Autodesk Fusion 360 part; units mm, degrees
(part 3 of 4)
sketch "草图57" plane through (0, 12.5, 0) normal (0, 1, 0) x (-1, 0, 0)
  circle A0 centre (-311.895, -3.8697) radius 1.7
  circle A1 centre (-109.895, -3.8697) radius 1.7
  circle A2 centre (-7.0941, -106.12) radius 1.7
  circle A3 centre (-7.0941, -3.8697) radius 1.7
  circle A4 centre (-210.895, -3.8697) radius 1.7
  circle A5 centre (-311.895, -106.12) radius 1.7
  circle A6 centre (-210.895, -106.12) radius 1.1
  circle A7 centre (-109.895, -106.12) radius 1.1
  arc A8 (-12.4713, -23.8643) -> (-11.9713, -23.3643) centre (-12.4713, -23.3643) ccw
  line L0 (-12.4713, -23.8643) -> (-25.4713, -23.8643)
  arc A9 (-25.9713, -23.3643) -> (-25.4713, -23.8643) centre (-25.4713, -23.3643) ccw
  line L1 (-25.9713, -23.3643) -> (-25.9713, -10.3643)
  arc A10 (-25.4713, -9.8643) -> (-25.9713, -10.3643) centre (-25.4713, -10.3643) ccw
  line L2 (-25.4713, -9.8643) -> (-12.4713, -9.8643)
  arc A11 (-11.9713, -10.3643) -> (-12.4713, -9.8643) centre (-12.4713, -10.3643) ccw
  line L3 (-11.9713, -10.3643) -> (-11.9713, -23.3643)
  arc A12 (-186.3026, -42.9143) -> (-185.8026, -42.4143) centre (-186.3026, -42.4143) ccw
  line L4 (-186.3026, -42.9143) -> (-199.3026, -42.9143)
  arc A13 (-199.8026, -42.4143) -> (-199.3026, -42.9143) centre (-199.3026, -42.4143) ccw
  line L5 (-199.8026, -42.4143) -> (-199.8026, -29.4143)
  arc A14 (-199.3026, -28.9143) -> (-199.8026, -29.4143) centre (-199.3026, -29.4143) ccw
  line L6 (-199.3026, -28.9143) -> (-186.3026, -28.9143)
  arc A15 (-185.8026, -29.4143) -> (-186.3026, -28.9143) centre (-186.3026, -29.4143) ccw
  line L7 (-185.8026, -29.4143) -> (-185.8026, -42.4143)
  arc A16 (-295.8401, -61.9643) -> (-295.3401, -61.4643) centre (-295.8401, -61.4643) ccw
  line L8 (-295.8401, -61.9643) -> (-308.8401, -61.9643)
  arc A17 (-309.3401, -61.4643) -> (-308.8401, -61.9643) centre (-308.8401, -61.4643) ccw
  line L9 (-309.3401, -61.4643) -> (-309.3401, -48.4643)
  arc A18 (-308.8401, -47.9643) -> (-309.3401, -48.4643) centre (-308.8401, -48.4643) ccw
  line L10 (-308.8401, -47.9643) -> (-295.8401, -47.9643)
  arc A19 (-295.3401, -48.4643) -> (-295.8401, -47.9643) centre (-295.8401, -48.4643) ccw
  line L11 (-295.3401, -48.4643) -> (-295.3401, -61.4643)
  line L12 (-128.6526, -29.4143) -> (-128.6526, -42.4143)
  arc A20 (-129.1526, -42.9143) -> (-128.6526, -42.4143) centre (-129.1526, -42.4143) ccw
  line L13 (-129.1526, -42.9143) -> (-142.1526, -42.9143)
  arc A21 (-142.6526, -42.4143) -> (-142.1526, -42.9143) centre (-142.1526, -42.4143) ccw
  line L14 (-142.6526, -42.4143) -> (-142.6526, -29.4143)
  arc A22 (-142.1526, -28.9143) -> (-142.6526, -29.4143) centre (-142.1526, -29.4143) ccw
  line L15 (-142.1526, -28.9143) -> (-129.1526, -28.9143)
  arc A23 (-128.6526, -29.4143) -> (-129.1526, -28.9143) centre (-129.1526, -29.4143) ccw
  arc A24 (-162.4901, -100.0643) -> (-161.9901, -99.5643) centre (-162.4901, -99.5643) ccw
  line L16 (-162.4901, -100.0643) -> (-175.4901, -100.0643)
  arc A25 (-175.9901, -99.5643) -> (-175.4901, -100.0643) centre (-175.4901, -99.5643) ccw
  line L17 (-175.9901, -99.5643) -> (-175.9901, -86.5643)
  arc A26 (-175.4901, -86.0643) -> (-175.9901, -86.5643) centre (-175.4901, -86.5643) ccw
  line L18 (-175.4901, -86.0643) -> (-162.4901, -86.0643)
  arc A27 (-161.9901, -86.5643) -> (-162.4901, -86.0643) centre (-162.4901, -86.5643) ccw
  line L19 (-161.9901, -86.5643) -> (-161.9901, -99.5643)
  arc A28 (-72.0026, -42.9143) -> (-71.5026, -42.4143) centre (-72.0026, -42.4143) ccw
  line L20 (-72.0026, -42.9143) -> (-85.0026, -42.9143)
  arc A29 (-85.5026, -42.4143) -> (-85.0026, -42.9143) centre (-85.0026, -42.4143) ccw
  line L21 (-85.5026, -42.4143) -> (-85.5026, -29.4143)
  arc A30 (-85.0026, -28.9143) -> (-85.5026, -29.4143) centre (-85.0026, -29.4143) ccw
  line L22 (-85.0026, -28.9143) -> (-72.0026, -28.9143)
  arc A31 (-71.5026, -29.4143) -> (-72.0026, -28.9143) centre (-72.0026, -29.4143) ccw
  line L23 (-71.5026, -29.4143) -> (-71.5026, -42.4143)
  arc A32 (-295.8401, -42.9143) -> (-295.3401, -42.4143) centre (-295.8401, -42.4143) ccw
  line L24 (-295.8401, -42.9143) -> (-308.8401, -42.9143)
  arc A33 (-309.3401, -42.4143) -> (-308.8401, -42.9143) centre (-308.8401, -42.4143) ccw
  line L25 (-309.3401, -42.4143) -> (-309.3401, -29.4143)
  arc A34 (-308.8401, -28.9143) -> (-309.3401, -29.4143) centre (-308.8401, -29.4143) ccw
  line L26 (-308.8401, -28.9143) -> (-295.8401, -28.9143)
  arc A35 (-295.3401, -29.4143) -> (-295.8401, -28.9143) centre (-295.8401, -29.4143) ccw
  line L27 (-295.3401, -29.4143) -> (-295.3401, -42.4143)
  arc A36 (-256.4458, -60.9643) -> (-255.9458, -60.4643) centre (-256.4458, -60.4643) ccw
  line L28 (-256.4458, -60.9643) -> (-262.4458, -60.9643)
  arc A37 (-262.9458, -60.4643) -> (-262.4458, -60.9643) centre (-262.4458, -60.4643) ccw
  line L29 (-262.9458, -60.4643) -> (-262.9458, -46.4643)
  arc A38 (-262.4458, -45.9643) -> (-262.9458, -46.4643) centre (-262.4458, -46.4643) ccw
  line L30 (-262.4458, -45.9643) -> (-256.4458, -45.9643)
  arc A39 (-255.9458, -46.4643) -> (-256.4458, -45.9643) centre (-256.4458, -46.4643) ccw
  line L31 (-255.9458, -46.4643) -> (-255.9458, -60.4643)
  arc A40 (-110.1026, -42.9143) -> (-109.6026, -42.4143) centre (-110.1026, -42.4143) ccw
  line L32 (-110.1026, -42.9143) -> (-123.1026, -42.9143)
  arc A41 (-123.6026, -42.4143) -> (-123.1026, -42.9143) centre (-123.1026, -42.4143) ccw
  line L33 (-123.6026, -42.4143) -> (-123.6026, -29.4143)
  arc A42 (-123.1026, -28.9143) -> (-123.6026, -29.4143) centre (-123.1026, -29.4143) ccw
  line L34 (-123.1026, -28.9143) -> (-110.1026, -28.9143)
  arc A43 (-109.6026, -29.4143) -> (-110.1026, -28.9143) centre (-110.1026, -29.4143) ccw
  line L35 (-109.6026, -29.4143) -> (-109.6026, -42.4143)
  line L36 (-52.4526, -29.4143) -> (-52.4526, -42.4143)
  arc A44 (-52.9526, -42.9143) -> (-52.4526, -42.4143) centre (-52.9526, -42.4143) ccw
  line L37 (-52.9526, -42.9143) -> (-65.9526, -42.9143)
  arc A45 (-66.4526, -42.4143) -> (-65.9526, -42.9143) centre (-65.9526, -42.4143) ccw
  line L38 (-66.4526, -42.4143) -> (-66.4526, -29.4143)
  arc A46 (-65.9526, -28.9143) -> (-66.4526, -29.4143) centre (-65.9526, -29.4143) ccw
  line L39 (-65.9526, -28.9143) -> (-52.9526, -28.9143)
  arc A47 (-52.4526, -29.4143) -> (-52.9526, -28.9143) centre (-52.9526, -29.4143) ccw
  arc A48 (-148.2026, -42.9143) -> (-147.7026, -42.4143) centre (-148.2026, -42.4143) ccw
  line L40 (-148.2026, -42.9143) -> (-161.2026, -42.9143)
  arc A49 (-161.7026, -42.4143) -> (-161.2026, -42.9143) centre (-161.2026, -42.4143) ccw
  line L41 (-161.7026, -42.4143) -> (-161.7026, -29.4143)
  arc A50 (-161.2026, -28.9143) -> (-161.7026, -29.4143) centre (-161.2026, -29.4143) ccw
  line L42 (-161.2026, -28.9143) -> (-148.2026, -28.9143)
  arc A51 (-147.7026, -29.4143) -> (-148.2026, -28.9143) centre (-148.2026, -29.4143) ccw
  line L43 (-147.7026, -29.4143) -> (-147.7026, -42.4143)
  arc A52 (-282.7031, -99.0643) -> (-282.2031, -98.5643) centre (-282.7031, -98.5643) ccw
  line L44 (-282.7031, -99.0643) -> (-288.7031, -99.0643)
  arc A53 (-289.2031, -98.5643) -> (-288.7031, -99.0643) centre (-288.7031, -98.5643) ccw
  line L45 (-289.2031, -98.5643) -> (-289.2031, -84.5643)
  arc A54 (-288.7031, -84.0643) -> (-289.2031, -84.5643) centre (-288.7031, -84.5643) ccw
  line L46 (-288.7031, -84.0643) -> (-282.7031, -84.0643)
  arc A55 (-282.2031, -84.5643) -> (-282.7031, -84.0643) centre (-282.7031, -84.5643) ccw
  line L47 (-282.2031, -84.5643) -> (-282.2031, -98.5643)
  arc A56 (-23.5901, -99.5643) -> (-23.0901, -100.0643) centre (-23.0901, -99.5643) ccw
  line L48 (-23.5901, -99.5643) -> (-23.5901, -86.5643)
  arc A57 (-23.0901, -86.0643) -> (-23.5901, -86.5643) centre (-23.0901, -86.5643) ccw
  line L49 (-23.0901, -86.0643) -> (-10.0901, -86.0643)
  arc A58 (-9.5901, -86.5643) -> (-10.0901, -86.0643) centre (-10.0901, -86.5643) ccw
  line L50 (-9.5901, -86.5643) -> (-9.5901, -99.5643)
  arc A59 (-10.0901, -100.0643) -> (-9.5901, -99.5643) centre (-10.0901, -99.5643) ccw
  line L51 (-10.0901, -100.0643) -> (-23.0901, -100.0643)
  arc A60 (-60.0963, -23.8643) -> (-59.5963, -23.3643) centre (-60.0963, -23.3643) ccw
  line L52 (-60.0963, -23.8643) -> (-73.0963, -23.8643)
  arc A61 (-73.5963, -23.3643) -> (-73.0963, -23.8643) centre (-73.0963, -23.3643) ccw
  line L53 (-73.5963, -23.3643) -> (-73.5963, -10.3643)
  arc A62 (-73.0963, -9.8643) -> (-73.5963, -10.3643) centre (-73.0963, -10.3643) ccw
  line L54 (-73.0963, -9.8643) -> (-60.0963, -9.8643)
  arc A63 (-59.5963, -10.3643) -> (-60.0963, -9.8643) centre (-60.0963, -10.3643) ccw
  line L55 (-59.5963, -10.3643) -> (-59.5963, -23.3643)
  arc A64 (-181.5401, -100.0643) -> (-181.0401, -99.5643) centre (-181.5401, -99.5643) ccw
  line L56 (-181.5401, -100.0643) -> (-194.5401, -100.0643)
  arc A65 (-195.0401, -99.5643) -> (-194.5401, -100.0643) centre (-194.5401, -99.5643) ccw
  line L57 (-195.0401, -99.5643) -> (-195.0401, -86.5643)
  arc A66 (-194.5401, -86.0643) -> (-195.0401, -86.5643) centre (-194.5401, -86.5643) ccw
  line L58 (-194.5401, -86.0643) -> (-181.5401, -86.0643)
  arc A67 (-181.0401, -86.5643) -> (-181.5401, -86.0643) centre (-181.5401, -86.5643) ccw
  line L59 (-181.0401, -86.5643) -> (-181.0401, -99.5643)
  arc A68 (-105.3401, -100.0643) -> (-104.8401, -99.5643) centre (-105.3401, -99.5643) ccw
  line L60 (-105.3401, -100.0643) -> (-118.3401, -100.0643)
  arc A69 (-118.8401, -99.5643) -> (-118.3401, -100.0643) centre (-118.3401, -99.5643) ccw
  line L61 (-118.8401, -99.5643) -> (-118.8401, -86.5643)
  arc A70 (-118.3401, -86.0643) -> (-118.8401, -86.5643) centre (-118.3401, -86.5643) ccw
  line L62 (-118.3401, -86.0643) -> (-105.3401, -86.0643)
  arc A71 (-104.8401, -86.5643) -> (-105.3401, -86.0643) centre (-105.3401, -86.5643) ccw
  line L63 (-104.8401, -86.5643) -> (-104.8401, -99.5643)
  arc A72 (-131.5338, -23.8643) -> (-131.0338, -23.3643) centre (-131.5338, -23.3643) ccw
  line L64 (-131.5338, -23.8643) -> (-144.5338, -23.8643)
  arc A73 (-145.0338, -23.3643) -> (-144.5338, -23.8643) centre (-144.5338, -23.3643) ccw
  line L65 (-145.0338, -23.3643) -> (-145.0338, -10.3643)
  arc A74 (-144.5338, -9.8643) -> (-145.0338, -10.3643) centre (-144.5338, -10.3643) ccw
  line L66 (-144.5338, -9.8643) -> (-131.5338, -9.8643)
  arc A75 (-131.0338, -10.3643) -> (-131.5338, -9.8643) centre (-131.5338, -10.3643) ccw
  line L67 (-131.0338, -10.3643) -> (-131.0338, -23.3643)
  arc A76 (-172.0151, -81.0143) -> (-171.5151, -80.5143) centre (-172.0151, -80.5143) ccw
  line L68 (-172.0151, -81.0143) -> (-185.0151, -81.0143)
  arc A77 (-185.5151, -80.5143) -> (-185.0151, -81.0143) centre (-185.0151, -80.5143) ccw
  line L69 (-185.5151, -80.5143) -> (-185.5151, -67.5143)
  arc A78 (-185.0151, -67.0143) -> (-185.5151, -67.5143) centre (-185.0151, -67.5143) ccw
  line L70 (-185.0151, -67.0143) -> (-172.0151, -67.0143)
  arc A79 (-171.5151, -67.5143) -> (-172.0151, -67.0143) centre (-172.0151, -67.5143) ccw
  line L71 (-171.5151, -67.5143) -> (-171.5151, -80.5143)
  arc A80 (-264.8838, -61.9643) -> (-264.3838, -61.4643) centre (-264.8838, -61.4643) ccw
  line L72 (-264.8838, -61.9643) -> (-277.8838, -61.9643)
  arc A81 (-278.3838, -61.4643) -> (-277.8838, -61.9643) centre (-277.8838, -61.4643) ccw
  line L73 (-278.3838, -61.4643) -> (-278.3838, -48.4643)
  arc A82 (-277.8838, -47.9643) -> (-278.3838, -48.4643) centre (-277.8838, -48.4643) ccw
  line L74 (-277.8838, -47.9643) -> (-264.8838, -47.9643)
  arc A83 (-264.3838, -48.4643) -> (-264.8838, -47.9643) centre (-264.8838, -48.4643) ccw
  line L75 (-264.3838, -48.4643) -> (-264.3838, -61.4643)
  arc A84 (-272.0276, -81.0143) -> (-271.5276, -80.5143) centre (-272.0276, -80.5143) ccw
  line L76 (-272.0276, -81.0143) -> (-285.0276, -81.0143)
  arc A85 (-285.5276, -80.5143) -> (-285.0276, -81.0143) centre (-285.0276, -80.5143) ccw
  line L77 (-285.5276, -80.5143) -> (-285.5276, -67.5143)
  arc A86 (-285.0276, -67.0143) -> (-285.5276, -67.5143) centre (-285.0276, -67.5143) ccw
  line L78 (-285.0276, -67.0143) -> (-272.0276, -67.0143)
  arc A87 (-271.5276, -67.5143) -> (-272.0276, -67.0143) centre (-272.0276, -67.5143) ccw
  line L79 (-271.5276, -67.5143) -> (-271.5276, -80.5143)
  line L80 (-157.2276, -48.4643) -> (-157.2276, -61.4643)
  arc A88 (-157.7276, -61.9643) -> (-157.2276, -61.4643) centre (-157.7276, -61.4643) ccw
  line L81 (-157.7276, -61.9643) -> (-170.7276, -61.9643)
  arc A89 (-171.2276, -61.4643) -> (-170.7276, -61.9643) centre (-170.7276, -61.4643) ccw
  line L82 (-171.2276, -61.4643) -> (-171.2276, -48.4643)
  arc A90 (-170.7276, -47.9643) -> (-171.2276, -48.4643) centre (-170.7276, -48.4643) ccw
  line L83 (-170.7276, -47.9643) -> (-157.7276, -47.9643)
  arc A91 (-157.2276, -48.4643) -> (-157.7276, -47.9643) centre (-157.7276, -48.4643) ccw
  arc A92 (-191.0651, -81.0143) -> (-190.5651, -80.5143) centre (-191.0651, -80.5143) ccw
  line L84 (-191.0651, -81.0143) -> (-204.0651, -81.0143)
  arc A93 (-204.5651, -80.5143) -> (-204.0651, -81.0143) centre (-204.0651, -80.5143) ccw
  line L85 (-204.5651, -80.5143) -> (-204.5651, -67.5143)
  arc A94 (-204.0651, -67.0143) -> (-204.5651, -67.5143) centre (-204.0651, -67.5143) ccw
  line L86 (-204.0651, -67.0143) -> (-191.0651, -67.0143)
  arc A95 (-190.5651, -67.5143) -> (-191.0651, -67.0143) centre (-191.0651, -67.5143) ccw
  line L87 (-190.5651, -67.5143) -> (-190.5651, -80.5143)
  arc A96 (-14.8526, -81.0143) -> (-14.3526, -80.5143) centre (-14.8526, -80.5143) ccw
  line L88 (-14.8526, -81.0143) -> (-27.8526, -81.0143)
  arc A97 (-28.3526, -80.5143) -> (-27.8526, -81.0143) centre (-27.8526, -80.5143) ccw
  line L89 (-28.3526, -80.5143) -> (-28.3526, -67.5143)
  arc A98 (-27.8526, -67.0143) -> (-28.3526, -67.5143) centre (-27.8526, -67.5143) ccw
  line L90 (-27.8526, -67.0143) -> (-14.8526, -67.0143)
  arc A99 (-14.3526, -67.5143) -> (-14.8526, -67.0143) centre (-14.8526, -67.5143) ccw
  line L91 (-14.3526, -67.5143) -> (-14.3526, -80.5143)
  arc A100 (-224.4026, -42.9143) -> (-223.9026, -42.4143) centre (-224.4026, -42.4143) ccw
  line L92 (-224.4026, -42.9143) -> (-237.4026, -42.9143)
  arc A101 (-237.9026, -42.4143) -> (-237.4026, -42.9143) centre (-237.4026, -42.4143) ccw
  line L93 (-237.9026, -42.4143) -> (-237.9026, -29.4143)
  arc A102 (-237.4026, -28.9143) -> (-237.9026, -29.4143) centre (-237.4026, -29.4143) ccw
  line L94 (-237.4026, -28.9143) -> (-224.4026, -28.9143)
  arc A103 (-223.9026, -29.4143) -> (-224.4026, -28.9143) centre (-224.4026, -29.4143) ccw
  line L95 (-223.9026, -29.4143) -> (-223.9026, -42.4143)
  arc A104 (-100.5776, -61.9643) -> (-100.0776, -61.4643) centre (-100.5776, -61.4643) ccw
  line L96 (-100.5776, -61.9643) -> (-113.5776, -61.9643)
  arc A105 (-114.0776, -61.4643) -> (-113.5776, -61.9643) centre (-113.5776, -61.4643) ccw
  line L97 (-114.0776, -61.4643) -> (-114.0776, -48.4643)
  arc A106 (-113.5776, -47.9643) -> (-114.0776, -48.4643) centre (-113.5776, -48.4643) ccw
  line L98 (-113.5776, -47.9643) -> (-100.5776, -47.9643)
  arc A107 (-100.0776, -48.4643) -> (-100.5776, -47.9643) centre (-100.5776, -48.4643) ccw
  line L99 (-100.0776, -48.4643) -> (-100.0776, -61.4643)
  arc A108 (-75.9776, -61.4643) -> (-75.4776, -61.9643) centre (-75.4776, -61.4643) ccw
  line L100 (-75.9776, -61.4643) -> (-75.9776, -48.4643)
  arc A109 (-75.4776, -47.9643) -> (-75.9776, -48.4643) centre (-75.4776, -48.4643) ccw
  line L101 (-75.4776, -47.9643) -> (-62.4776, -47.9643)
  arc A110 (-61.9776, -48.4643) -> (-62.4776, -47.9643) centre (-62.4776, -48.4643) ccw
  line L102 (-61.9776, -48.4643) -> (-61.9776, -61.4643)
  arc A111 (-62.4776, -61.9643) -> (-61.9776, -61.4643) centre (-62.4776, -61.4643) ccw
  line L103 (-62.4776, -61.9643) -> (-75.4776, -61.9643)
  line L104 (-142.9401, -86.5643) -> (-142.9401, -99.5643)
  arc A112 (-143.4401, -100.0643) -> (-142.9401, -99.5643) centre (-143.4401, -99.5643) ccw
  line L105 (-143.4401, -100.0643) -> (-156.4401, -100.0643)
  arc A113 (-156.9401, -99.5643) -> (-156.4401, -100.0643) centre (-156.4401, -99.5643) ccw
  line L106 (-156.9401, -99.5643) -> (-156.9401, -86.5643)
  arc A114 (-156.4401, -86.0643) -> (-156.9401, -86.5643) centre (-156.4401, -86.5643) ccw
  line L107 (-156.4401, -86.0643) -> (-143.4401, -86.0643)
  arc A115 (-142.9401, -86.5643) -> (-143.4401, -86.0643) centre (-143.4401, -86.5643) ccw
  arc A116 (-202.9713, -23.8643) -> (-202.4713, -23.3643) centre (-202.9713, -23.3643) ccw
  line L108 (-202.9713, -23.8643) -> (-215.9713, -23.8643)
  arc A117 (-216.4713, -23.3643) -> (-215.9713, -23.8643) centre (-215.9713, -23.3643) ccw
  line L109 (-216.4713, -23.3643) -> (-216.4713, -10.3643)
  arc A118 (-215.9713, -9.8643) -> (-216.4713, -10.3643) centre (-215.9713, -10.3643) ccw
  line L110 (-215.9713, -9.8643) -> (-202.9713, -9.8643)
  arc A119 (-202.4713, -10.3643) -> (-202.9713, -9.8643) centre (-202.9713, -10.3643) ccw
  line L111 (-202.4713, -10.3643) -> (-202.4713, -23.3643)
  arc A120 (-185.0338, -22.8643) -> (-184.5338, -22.3643) centre (-185.0338, -22.3643) ccw
  line L112 (-185.0338, -22.8643) -> (-191.0338, -22.8643)
  arc A121 (-191.5338, -22.3643) -> (-191.0338, -22.8643) centre (-191.0338, -22.3643) ccw
  line L113 (-191.5338, -22.3643) -> (-191.5338, -8.3643)
  arc A122 (-191.0338, -7.8643) -> (-191.5338, -8.3643) centre (-191.0338, -8.3643) ccw
  line L114 (-191.0338, -7.8643) -> (-185.0338, -7.8643)
  arc A123 (-184.5338, -8.3643) -> (-185.0338, -7.8643) centre (-185.0338, -8.3643) ccw
  line L115 (-184.5338, -8.3643) -> (-184.5338, -22.3643)
  arc A124 (-219.6401, -100.0643) -> (-219.1401, -99.5643) centre (-219.6401, -99.5643) ccw
  line L116 (-219.6401, -100.0643) -> (-232.6401, -100.0643)
  arc A125 (-233.1401, -99.5643) -> (-232.6401, -100.0643) centre (-232.6401, -99.5643) ccw
  line L117 (-233.1401, -99.5643) -> (-233.1401, -86.5643)
  arc A126 (-232.6401, -86.0643) -> (-233.1401, -86.5643) centre (-232.6401, -86.5643) ccw
  line L118 (-232.6401, -86.0643) -> (-219.6401, -86.0643)
  arc A127 (-219.1401, -86.5643) -> (-219.6401, -86.0643) centre (-219.6401, -86.5643) ccw
  line L119 (-219.1401, -86.5643) -> (-219.1401, -99.5643)
  arc A128 (-76.7651, -81.0143) -> (-76.2651, -80.5143) centre (-76.7651, -80.5143) ccw
  line L120 (-76.7651, -81.0143) -> (-89.7651, -81.0143)
  arc A129 (-90.2651, -80.5143) -> (-89.7651, -81.0143) centre (-89.7651, -80.5143) ccw
  line L121 (-90.2651, -80.5143) -> (-90.2651, -67.5143)
  arc A130 (-89.7651, -67.0143) -> (-90.2651, -67.5143) centre (-89.7651, -67.5143) ccw
  line L122 (-89.7651, -67.0143) -> (-76.7651, -67.0143)
  arc A131 (-76.2651, -67.5143) -> (-76.7651, -67.0143) centre (-76.7651, -67.5143) ccw
  line L123 (-76.2651, -67.5143) -> (-76.2651, -80.5143)
  line L124 (-166.7526, -29.4143) -> (-166.7526, -42.4143)
  arc A132 (-167.2526, -42.9143) -> (-166.7526, -42.4143) centre (-167.2526, -42.4143) ccw
  line L125 (-167.2526, -42.9143) -> (-180.2526, -42.9143)
  arc A133 (-180.7526, -42.4143) -> (-180.2526, -42.9143) centre (-180.2526, -42.4143) ccw
  line L126 (-180.7526, -42.4143) -> (-180.7526, -29.4143)
  arc A134 (-180.2526, -28.9143) -> (-180.7526, -29.4143) centre (-180.2526, -29.4143) ccw
  line L127 (-180.2526, -28.9143) -> (-167.2526, -28.9143)
  arc A135 (-166.7526, -29.4143) -> (-167.2526, -28.9143) centre (-167.2526, -29.4143) ccw
  arc A136 (-152.9651, -81.0143) -> (-152.4651, -80.5143) centre (-152.9651, -80.5143) ccw
  line L128 (-152.9651, -81.0143) -> (-165.9651, -81.0143)
  arc A137 (-166.4651, -80.5143) -> (-165.9651, -81.0143) centre (-165.9651, -80.5143) ccw
  line L129 (-166.4651, -80.5143) -> (-166.4651, -67.5143)
  arc A138 (-165.9651, -67.0143) -> (-166.4651, -67.5143) centre (-165.9651, -67.5143) ccw
  line L130 (-165.9651, -67.0143) -> (-152.9651, -67.0143)
  arc A139 (-152.4651, -67.5143) -> (-152.9651, -67.0143) centre (-152.9651, -67.5143) ccw
  line L131 (-152.4651, -67.5143) -> (-152.4651, -80.5143)
  line L132 (-209.6151, -67.5143) -> (-209.6151, -80.5143)
  arc A140 (-210.1151, -81.0143) -> (-209.6151, -80.5143) centre (-210.1151, -80.5143) ccw
  line L133 (-210.1151, -81.0143) -> (-223.1151, -81.0143)
  arc A141 (-223.6151, -80.5143) -> (-223.1151, -81.0143) centre (-223.1151, -80.5143) ccw
  line L134 (-223.6151, -80.5143) -> (-223.6151, -67.5143)
  arc A142 (-223.1151, -67.0143) -> (-223.6151, -67.5143) centre (-223.1151, -67.5143) ccw
  line L135 (-223.1151, -67.0143) -> (-210.1151, -67.0143)
  arc A143 (-209.6151, -67.5143) -> (-210.1151, -67.0143) centre (-210.1151, -67.5143) ccw
  arc A144 (-257.7401, -23.8643) -> (-257.2401, -23.3643) centre (-257.7401, -23.3643) ccw
  line L136 (-257.7401, -23.8643) -> (-270.7401, -23.8643)
  arc A145 (-271.2401, -23.3643) -> (-270.7401, -23.8643) centre (-270.7401, -23.3643) ccw
  line L137 (-271.2401, -23.3643) -> (-271.2401, -10.3643)
  arc A146 (-270.7401, -9.8643) -> (-271.2401, -10.3643) centre (-270.7401, -10.3643) ccw
  line L138 (-270.7401, -9.8643) -> (-257.7401, -9.8643)
  arc A147 (-257.2401, -10.3643) -> (-257.7401, -9.8643) centre (-257.7401, -10.3643) ccw
  line L139 (-257.2401, -10.3643) -> (-257.2401, -23.3643)
  arc A148 (-250.5963, -42.9143) -> (-250.0963, -42.4143) centre (-250.5963, -42.4143) ccw
  line L140 (-250.5963, -42.9143) -> (-263.5963, -42.9143)
  arc A149 (-264.0963, -42.4143) -> (-263.5963, -42.9143) centre (-263.5963, -42.4143) ccw
  line L141 (-264.0963, -42.4143) -> (-264.0963, -29.4143)
  arc A150 (-263.5963, -28.9143) -> (-264.0963, -29.4143) centre (-263.5963, -29.4143) ccw
  line L142 (-263.5963, -28.9143) -> (-250.5963, -28.9143)
  arc A151 (-250.0963, -29.4143) -> (-250.5963, -28.9143) centre (-250.5963, -29.4143) ccw
  line L143 (-250.0963, -29.4143) -> (-250.0963, -42.4143)
  arc A152 (-21.9963, -42.9143) -> (-21.4963, -42.4143) centre (-21.9963, -42.4143) ccw
  line L144 (-21.9963, -42.9143) -> (-34.9963, -42.9143)
  arc A153 (-35.4963, -42.4143) -> (-34.9963, -42.9143) centre (-34.9963, -42.4143) ccw
  line L145 (-35.4963, -42.4143) -> (-35.4963, -29.4143)
  arc A154 (-34.9963, -28.9143) -> (-35.4963, -29.4143) centre (-34.9963, -29.4143) ccw
  line L146 (-34.9963, -28.9143) -> (-21.9963, -28.9143)
  arc A155 (-21.4963, -29.4143) -> (-21.9963, -28.9143) centre (-21.9963, -29.4143) ccw
  line L147 (-21.4963, -29.4143) -> (-21.4963, -42.4143)
  arc A156 (-48.1901, -100.0643) -> (-47.6901, -99.5643) centre (-48.1901, -99.5643) ccw
  line L148 (-48.1901, -100.0643) -> (-61.1901, -100.0643)
  arc A157 (-61.6901, -99.5643) -> (-61.1901, -100.0643) centre (-61.1901, -99.5643) ccw
  line L149 (-61.6901, -99.5643) -> (-61.6901, -86.5643)
  arc A158 (-61.1901, -86.0643) -> (-61.6901, -86.5643) centre (-61.1901, -86.5643) ccw
  line L150 (-61.1901, -86.0643) -> (-48.1901, -86.0643)
  arc A159 (-47.6901, -86.5643) -> (-48.1901, -86.0643) centre (-48.1901, -86.5643) ccw
  line L151 (-47.6901, -86.5643) -> (-47.6901, -99.5643)
  arc A160 (-280.3218, -60.9643) -> (-279.8218, -60.4643) centre (-280.3218, -60.4643) ccw
  line L152 (-280.3218, -60.9643) -> (-286.3218, -60.9643)
  arc A161 (-286.8218, -60.4643) -> (-286.3218, -60.9643) centre (-286.3218, -60.4643) ccw
  line L153 (-286.8218, -60.4643) -> (-286.8218, -46.4643)
  arc A162 (-286.3218, -45.9643) -> (-286.8218, -46.4643) centre (-286.3218, -46.4643) ccw
  line L154 (-286.3218, -45.9643) -> (-280.3218, -45.9643)
  arc A163 (-279.8218, -46.4643) -> (-280.3218, -45.9643) centre (-280.3218, -46.4643) ccw
  line L155 (-279.8218, -46.4643) -> (-279.8218, -60.4643)
  line L156 (-84.5338, -8.3643) -> (-84.5338, -22.3643)
  arc A164 (-85.0338, -22.8643) -> (-84.5338, -22.3643) centre (-85.0338, -22.3643) ccw
  line L157 (-85.0338, -22.8643) -> (-91.0338, -22.8643)
  arc A165 (-91.5338, -22.3643) -> (-91.0338, -22.8643) centre (-91.0338, -22.3643) ccw
  line L158 (-91.5338, -22.3643) -> (-91.5338, -8.3643)
  arc A166 (-91.0338, -7.8643) -> (-91.5338, -8.3643) centre (-91.0338, -8.3643) ccw
  line L159 (-91.0338, -7.8643) -> (-85.0338, -7.8643)
  arc A167 (-84.5338, -8.3643) -> (-85.0338, -7.8643) centre (-85.0338, -8.3643) ccw
  arc A168 (-233.9276, -61.9643) -> (-233.4276, -61.4643) centre (-233.9276, -61.4643) ccw
  line L160 (-233.9276, -61.9643) -> (-246.9276, -61.9643)
  arc A169 (-247.4276, -61.4643) -> (-246.9276, -61.9643) centre (-246.9276, -61.4643) ccw
  line L161 (-247.4276, -61.4643) -> (-247.4276, -48.4643)
  arc A170 (-246.9276, -47.9643) -> (-247.4276, -48.4643) centre (-246.9276, -48.4643) ccw
  line L162 (-246.9276, -47.9643) -> (-233.9276, -47.9643)
  arc A171 (-233.4276, -48.4643) -> (-233.9276, -47.9643) centre (-233.9276, -48.4643) ccw
  line L163 (-233.4276, -48.4643) -> (-233.4276, -61.4643)
  arc A172 (-119.6276, -61.9643) -> (-119.1276, -61.4643) centre (-119.6276, -61.4643) ccw
  line L164 (-119.6276, -61.9643) -> (-132.6276, -61.9643)
  arc A173 (-133.1276, -61.4643) -> (-132.6276, -61.9643) centre (-132.6276, -61.4643) ccw
  line L165 (-133.1276, -61.4643) -> (-133.1276, -48.4643)
  arc A174 (-132.6276, -47.9643) -> (-133.1276, -48.4643) centre (-132.6276, -48.4643) ccw
  line L166 (-132.6276, -47.9643) -> (-119.6276, -47.9643)
  arc A175 (-119.1276, -48.4643) -> (-119.6276, -47.9643) centre (-119.6276, -48.4643) ccw
  line L167 (-119.1276, -48.4643) -> (-119.1276, -61.4643)
  line L168 (-176.2776, -48.4643) -> (-176.2776, -61.4643)
  arc A176 (-176.7776, -61.9643) -> (-176.2776, -61.4643) centre (-176.7776, -61.4643) ccw
  line L169 (-176.7776, -61.9643) -> (-189.7776, -61.9643)
  arc A177 (-190.2776, -61.4643) -> (-189.7776, -61.9643) centre (-189.7776, -61.4643) ccw
  line L170 (-190.2776, -61.4643) -> (-190.2776, -48.4643)
  arc A178 (-189.7776, -47.9643) -> (-190.2776, -48.4643) centre (-189.7776, -48.4643) ccw
  line L171 (-189.7776, -47.9643) -> (-176.7776, -47.9643)
  arc A179 (-176.2776, -48.4643) -> (-176.7776, -47.9643) centre (-176.7776, -48.4643) ccw
  arc A180 (-214.8776, -61.9643) -> (-214.3776, -61.4643) centre (-214.8776, -61.4643) ccw
  line L172 (-214.8776, -61.9643) -> (-227.8776, -61.9643)
  arc A181 (-228.3776, -61.4643) -> (-227.8776, -61.9643) centre (-227.8776, -61.4643) ccw
  line L173 (-228.3776, -61.4643) -> (-228.3776, -48.4643)
  arc A182 (-227.8776, -47.9643) -> (-228.3776, -48.4643) centre (-227.8776, -48.4643) ccw
  line L174 (-227.8776, -47.9643) -> (-214.8776, -47.9643)
  arc A183 (-214.3776, -48.4643) -> (-214.8776, -47.9643) centre (-214.8776, -48.4643) ccw
  line L175 (-214.3776, -48.4643) -> (-214.3776, -61.4643)
  arc A184 (-276.7901, -42.9143) -> (-276.2901, -42.4143) centre (-276.7901, -42.4143) ccw
  line L176 (-276.7901, -42.9143) -> (-289.7901, -42.9143)
  arc A185 (-290.2901, -42.4143) -> (-289.7901, -42.9143) centre (-289.7901, -42.4143) ccw
  line L177 (-290.2901, -42.4143) -> (-290.2901, -29.4143)
  arc A186 (-289.7901, -28.9143) -> (-290.2901, -29.4143) centre (-289.7901, -29.4143) ccw
  line L178 (-289.7901, -28.9143) -> (-276.7901, -28.9143)
  arc A187 (-276.2901, -29.4143) -> (-276.7901, -28.9143) centre (-276.7901, -29.4143) ccw
  line L179 (-276.2901, -29.4143) -> (-276.2901, -42.4143)
  arc A188 (-114.8651, -81.0143) -> (-114.3651, -80.5143) centre (-114.8651, -80.5143) ccw
  line L180 (-114.8651, -81.0143) -> (-127.8651, -81.0143)
  arc A189 (-128.3651, -80.5143) -> (-127.8651, -81.0143) centre (-127.8651, -80.5143) ccw
  line L181 (-128.3651, -80.5143) -> (-128.3651, -67.5143)
  arc A190 (-127.8651, -67.0143) -> (-128.3651, -67.5143) centre (-127.8651, -67.5143) ccw
  line L182 (-127.8651, -67.0143) -> (-114.8651, -67.0143)
  arc A191 (-114.3651, -67.5143) -> (-114.8651, -67.0143) centre (-114.8651, -67.5143) ccw
  line L183 (-114.3651, -67.5143) -> (-114.3651, -80.5143)
  arc A192 (-124.3901, -100.0643) -> (-123.8901, -99.5643) centre (-124.3901, -99.5643) ccw
  line L184 (-124.3901, -100.0643) -> (-137.3901, -100.0643)
  arc A193 (-137.8901, -99.5643) -> (-137.3901, -100.0643) centre (-137.3901, -99.5643) ccw
  line L185 (-137.8901, -99.5643) -> (-137.8901, -86.5643)
  arc A194 (-137.3901, -86.0643) -> (-137.8901, -86.5643) centre (-137.3901, -86.5643) ccw
  line L186 (-137.3901, -86.0643) -> (-124.3901, -86.0643)
  arc A195 (-123.8901, -86.5643) -> (-124.3901, -86.0643) centre (-124.3901, -86.5643) ccw
  line L187 (-123.8901, -86.5643) -> (-123.8901, -99.5643)
  arc A196 (-57.7151, -81.0143) -> (-57.2151, -80.5143) centre (-57.7151, -80.5143) ccw
  line L188 (-57.7151, -81.0143) -> (-70.7151, -81.0143)
  arc A197 (-71.2151, -80.5143) -> (-70.7151, -81.0143) centre (-70.7151, -80.5143) ccw
  line L189 (-71.2151, -80.5143) -> (-71.2151, -67.5143)
  arc A198 (-70.7151, -67.0143) -> (-71.2151, -67.5143) centre (-70.7151, -67.5143) ccw
  line L190 (-70.7151, -67.0143) -> (-57.7151, -67.0143)
  arc A199 (-57.2151, -67.5143) -> (-57.7151, -67.0143) centre (-57.7151, -67.5143) ccw
  line L191 (-57.2151, -67.5143) -> (-57.2151, -80.5143)
  arc A200 (-29.1401, -100.0643) -> (-28.6401, -99.5643) centre (-29.1401, -99.5643) ccw
  line L192 (-29.1401, -100.0643) -> (-42.1401, -100.0643)
  arc A201 (-42.6401, -99.5643) -> (-42.1401, -100.0643) centre (-42.1401, -99.5643) ccw
  line L193 (-42.6401, -99.5643) -> (-42.6401, -86.5643)
  arc A202 (-42.1401, -86.0643) -> (-42.6401, -86.5643) centre (-42.1401, -86.5643) ccw
  line L194 (-42.1401, -86.0643) -> (-29.1401, -86.0643)
  arc A203 (-28.6401, -86.5643) -> (-29.1401, -86.0643) centre (-29.1401, -86.5643) ccw
  line L195 (-28.6401, -86.5643) -> (-28.6401, -99.5643)
  arc A204 (-295.8401, -23.8643) -> (-295.3401, -23.3643) centre (-295.8401, -23.3643) ccw
  line L196 (-295.8401, -23.8643) -> (-308.8401, -23.8643)
  arc A205 (-309.3401, -23.3643) -> (-308.8401, -23.8643) centre (-308.8401, -23.3643) ccw
  line L197 (-309.3401, -23.3643) -> (-309.3401, -10.3643)
  arc A206 (-308.8401, -9.8643) -> (-309.3401, -10.3643) centre (-308.8401, -10.3643) ccw
  line L198 (-308.8401, -9.8643) -> (-295.8401, -9.8643)
  arc A207 (-295.3401, -10.3643) -> (-295.8401, -9.8643) centre (-295.8401, -10.3643) ccw
  line L199 (-295.3401, -10.3643) -> (-295.3401, -23.3643)
  arc A208 (-248.2151, -81.0143) -> (-247.7151, -80.5143) centre (-248.2151, -80.5143) ccw
  line L200 (-248.2151, -81.0143) -> (-261.2151, -81.0143)
  arc A209 (-261.7151, -80.5143) -> (-261.2151, -81.0143) centre (-261.2151, -80.5143) ccw
  line L201 (-261.7151, -80.5143) -> (-261.7151, -67.5143)
  arc A210 (-261.2151, -67.0143) -> (-261.7151, -67.5143) centre (-261.2151, -67.5143) ccw
  line L202 (-261.2151, -67.0143) -> (-248.2151, -67.0143)
  arc A211 (-247.7151, -67.5143) -> (-248.2151, -67.0143) centre (-248.2151, -67.5143) ccw
  line L203 (-247.7151, -67.5143) -> (-247.7151, -80.5143)
  arc A212 (-67.2401, -100.0643) -> (-66.7401, -99.5643) centre (-67.2401, -99.5643) ccw
  line L204 (-67.2401, -100.0643) -> (-80.2401, -100.0643)
  arc A213 (-80.7401, -99.5643) -> (-80.2401, -100.0643) centre (-80.2401, -99.5643) ccw
  line L205 (-80.7401, -99.5643) -> (-80.7401, -86.5643)
  arc A214 (-80.2401, -86.0643) -> (-80.7401, -86.5643) centre (-80.2401, -86.5643) ccw
  line L206 (-80.2401, -86.0643) -> (-67.2401, -86.0643)
  arc A215 (-66.7401, -86.5643) -> (-67.2401, -86.0643) centre (-67.2401, -86.5643) ccw
  line L207 (-66.7401, -86.5643) -> (-66.7401, -99.5643)
  arc A216 (-200.5901, -100.0643) -> (-200.0901, -99.5643) centre (-200.5901, -99.5643) ccw
  line L208 (-200.5901, -100.0643) -> (-213.5901, -100.0643)
  arc A217 (-214.0901, -99.5643) -> (-213.5901, -100.0643) centre (-213.5901, -99.5643) ccw
  line L209 (-214.0901, -99.5643) -> (-214.0901, -86.5643)
  arc A218 (-213.5901, -86.0643) -> (-214.0901, -86.5643) centre (-213.5901, -86.5643) ccw
  line L210 (-213.5901, -86.0643) -> (-200.5901, -86.0643)
  arc A219 (-200.0901, -86.5643) -> (-200.5901, -86.0643) centre (-200.5901, -86.5643) ccw
  line L211 (-200.0901, -86.5643) -> (-200.0901, -99.5643)
  arc A220 (-95.0276, -61.4643) -> (-94.5276, -61.9643) centre (-94.5276, -61.4643) ccw
  line L212 (-95.0276, -61.4643) -> (-95.0276, -48.4643)
  arc A221 (-94.5276, -47.9643) -> (-95.0276, -48.4643) centre (-94.5276, -48.4643) ccw
  line L213 (-94.5276, -47.9643) -> (-81.5276, -47.9643)
  arc A222 (-81.0276, -48.4643) -> (-81.5276, -47.9643) centre (-81.5276, -48.4643) ccw
  line L214 (-81.0276, -48.4643) -> (-81.0276, -61.4643)
  arc A223 (-81.5276, -61.9643) -> (-81.0276, -61.4643) centre (-81.5276, -61.4643) ccw
  line L215 (-81.5276, -61.9643) -> (-94.5276, -61.9643)
  arc A224 (-295.8401, -81.0143) -> (-295.3401, -80.5143) centre (-295.8401, -80.5143) ccw
  line L216 (-295.8401, -81.0143) -> (-308.8401, -81.0143)
  arc A225 (-309.3401, -80.5143) -> (-308.8401, -81.0143) centre (-308.8401, -80.5143) ccw
  line L217 (-309.3401, -80.5143) -> (-309.3401, -67.5143)
  arc A226 (-308.8401, -67.0143) -> (-309.3401, -67.5143) centre (-308.8401, -67.5143) ccw
  line L218 (-308.8401, -67.0143) -> (-295.8401, -67.0143)
  arc A227 (-295.3401, -67.5143) -> (-295.8401, -67.0143) centre (-295.8401, -67.5143) ccw
  line L219 (-295.3401, -67.5143) -> (-295.3401, -80.5143)
  arc A228 (-205.3526, -42.9143) -> (-204.8526, -42.4143) centre (-205.3526, -42.4143) ccw
  line L220 (-205.3526, -42.9143) -> (-218.3526, -42.9143)
  arc A229 (-218.8526, -42.4143) -> (-218.3526, -42.9143) centre (-218.3526, -42.4143) ccw
  line L221 (-218.8526, -42.4143) -> (-218.8526, -29.4143)
  arc A230 (-218.3526, -28.9143) -> (-218.8526, -29.4143) centre (-218.3526, -29.4143) ccw
  line L222 (-218.3526, -28.9143) -> (-205.3526, -28.9143)
  arc A231 (-204.8526, -29.4143) -> (-205.3526, -28.9143) centre (-205.3526, -29.4143) ccw
  line L223 (-204.8526, -29.4143) -> (-204.8526, -42.4143)
  arc A232 (-36.2838, -23.8643) -> (-35.7838, -23.3643) centre (-36.2838, -23.3643) ccw
  line L224 (-36.2838, -23.8643) -> (-49.2838, -23.8643)
  arc A233 (-49.7838, -23.3643) -> (-49.2838, -23.8643) centre (-49.2838, -23.3643) ccw
  line L225 (-49.7838, -23.3643) -> (-49.7838, -10.3643)
  arc A234 (-49.2838, -9.8643) -> (-49.7838, -10.3643) centre (-49.2838, -10.3643) ccw
  line L226 (-49.2838, -9.8643) -> (-36.2838, -9.8643)
  arc A235 (-35.7838, -10.3643) -> (-36.2838, -9.8643) centre (-36.2838, -10.3643) ccw
  line L227 (-35.7838, -10.3643) -> (-35.7838, -23.3643)
  arc A236 (-43.4276, -61.9643) -> (-42.9276, -61.4643) centre (-43.4276, -61.4643) ccw
  line L228 (-43.4276, -61.9643) -> (-56.4276, -61.9643)
  arc A237 (-56.9276, -61.4643) -> (-56.4276, -61.9643) centre (-56.4276, -61.4643) ccw
  line L229 (-56.9276, -61.4643) -> (-56.9276, -48.4643)
  arc A238 (-56.4276, -47.9643) -> (-56.9276, -48.4643) centre (-56.4276, -48.4643) ccw
  line L230 (-56.4276, -47.9643) -> (-43.4276, -47.9643)
  arc A239 (-42.9276, -48.4643) -> (-43.4276, -47.9643) centre (-43.4276, -48.4643) ccw
  line L231 (-42.9276, -48.4643) -> (-42.9276, -61.4643)
  arc A240 (-52.1651, -80.5143) -> (-51.6651, -81.0143) centre (-51.6651, -80.5143) ccw
  line L232 (-52.1651, -80.5143) -> (-52.1651, -67.5143)
  arc A241 (-51.6651, -67.0143) -> (-52.1651, -67.5143) centre (-51.6651, -67.5143) ccw
  line L233 (-51.6651, -67.0143) -> (-38.6651, -67.0143)
  arc A242 (-38.1651, -67.5143) -> (-38.6651, -67.0143) centre (-38.6651, -67.5143) ccw
  line L234 (-38.1651, -67.5143) -> (-38.1651, -80.5143)
  arc A243 (-38.6651, -81.0143) -> (-38.1651, -80.5143) centre (-38.6651, -80.5143) ccw
  line L235 (-38.6651, -81.0143) -> (-51.6651, -81.0143)
  line L236 (-85.7901, -86.5643) -> (-85.7901, -99.5643)
  arc A244 (-86.2901, -100.0643) -> (-85.7901, -99.5643) centre (-86.2901, -99.5643) ccw
  line L237 (-86.2901, -100.0643) -> (-99.2901, -100.0643)
  arc A245 (-99.7901, -99.5643) -> (-99.2901, -100.0643) centre (-99.2901, -99.5643) ccw
  line L238 (-99.7901, -99.5643) -> (-99.7901, -86.5643)
  arc A246 (-99.2901, -86.0643) -> (-99.7901, -86.5643) centre (-99.2901, -86.5643) ccw
  line L239 (-99.2901, -86.0643) -> (-86.2901, -86.0643)
  arc A247 (-85.7901, -86.5643) -> (-86.2901, -86.0643) centre (-86.2901, -86.5643) ccw
  arc A248 (-276.7901, -23.8643) -> (-276.2901, -23.3643) centre (-276.7901, -23.3643) ccw
  line L240 (-276.7901, -23.8643) -> (-289.7901, -23.8643)
  arc A249 (-290.2901, -23.3643) -> (-289.7901, -23.8643) centre (-289.7901, -23.3643) ccw
  line L241 (-290.2901, -23.3643) -> (-290.2901, -10.3643)
  arc A250 (-289.7901, -9.8643) -> (-290.2901, -10.3643) centre (-289.7901, -10.3643) ccw
  line L242 (-289.7901, -9.8643) -> (-276.7901, -9.8643)
  arc A251 (-276.2901, -10.3643) -> (-276.7901, -9.8643) centre (-276.7901, -10.3643) ccw
  line L243 (-276.2901, -10.3643) -> (-276.2901, -23.3643)
  arc A252 (-13.5583, -41.9143) -> (-13.0583, -41.4143) centre (-13.5583, -41.4143) ccw
  line L244 (-13.5583, -41.9143) -> (-19.5583, -41.9143)
  arc A253 (-20.0583, -41.4143) -> (-19.5583, -41.9143) centre (-19.5583, -41.4143) ccw
  line L245 (-20.0583, -41.4143) -> (-20.0583, -27.4143)
  arc A254 (-19.5583, -26.9143) -> (-20.0583, -27.4143) centre (-19.5583, -27.4143) ccw
  line L246 (-19.5583, -26.9143) -> (-13.5583, -26.9143)
  arc A255 (-13.0583, -27.4143) -> (-13.5583, -26.9143) centre (-13.5583, -27.4143) ccw
  line L247 (-13.0583, -27.4143) -> (-13.0583, -41.4143)
  arc A256 (-226.7838, -23.8643) -> (-226.2838, -23.3643) centre (-226.7838, -23.3643) ccw
  line L248 (-226.7838, -23.8643) -> (-239.7838, -23.8643)
  arc A257 (-240.2838, -23.3643) -> (-239.7838, -23.8643) centre (-239.7838, -23.3643) ccw
  line L249 (-240.2838, -23.3643) -> (-240.2838, -10.3643)
  arc A258 (-239.7838, -9.8643) -> (-240.2838, -10.3643) centre (-239.7838, -10.3643) ccw
  line L250 (-239.7838, -9.8643) -> (-226.7838, -9.8643)
  arc A259 (-226.2838, -10.3643) -> (-226.7838, -9.8643) centre (-226.7838, -10.3643) ccw
  line L251 (-226.2838, -10.3643) -> (-226.2838, -23.3643)
  line L252 (-195.3276, -48.4643) -> (-195.3276, -61.4643)
  arc A260 (-195.8276, -61.9643) -> (-195.3276, -61.4643) centre (-195.8276, -61.4643) ccw
  line L253 (-195.8276, -61.9643) -> (-208.8276, -61.9643)
  arc A261 (-209.3276, -61.4643) -> (-208.8276, -61.9643) centre (-208.8276, -61.4643) ccw
  line L254 (-209.3276, -61.4643) -> (-209.3276, -48.4643)
  arc A262 (-208.8276, -47.9643) -> (-209.3276, -48.4643) centre (-208.8276, -48.4643) ccw
  line L255 (-208.8276, -47.9643) -> (-195.8276, -47.9643)
  arc A263 (-195.3276, -48.4643) -> (-195.8276, -47.9643) centre (-195.8276, -48.4643) ccw
  arc A264 (-229.1651, -81.0143) -> (-228.6651, -80.5143) centre (-229.1651, -80.5143) ccw
  line L256 (-229.1651, -81.0143) -> (-242.1651, -81.0143)
  arc A265 (-242.6651, -80.5143) -> (-242.1651, -81.0143) centre (-242.1651, -80.5143) ccw
  line L257 (-242.6651, -80.5143) -> (-242.6651, -67.5143)
  arc A266 (-242.1651, -67.0143) -> (-242.6651, -67.5143) centre (-242.1651, -67.5143) ccw
  line L258 (-242.1651, -67.0143) -> (-229.1651, -67.0143)
  arc A267 (-228.6651, -67.5143) -> (-229.1651, -67.0143) centre (-229.1651, -67.5143) ccw
  line L259 (-228.6651, -67.5143) -> (-228.6651, -80.5143)
  arc A268 (-91.0526, -42.9143) -> (-90.5526, -42.4143) centre (-91.0526, -42.4143) ccw
  line L260 (-91.0526, -42.9143) -> (-104.0526, -42.9143)
  arc A269 (-104.5526, -42.4143) -> (-104.0526, -42.9143) centre (-104.0526, -42.4143) ccw
  line L261 (-104.5526, -42.4143) -> (-104.5526, -29.4143)
  arc A270 (-104.0526, -28.9143) -> (-104.5526, -29.4143) centre (-104.0526, -29.4143) ccw
  line L262 (-104.0526, -28.9143) -> (-91.0526, -28.9143)
  arc A271 (-90.5526, -29.4143) -> (-91.0526, -28.9143) centre (-91.0526, -29.4143) ccw
  line L263 (-90.5526, -29.4143) -> (-90.5526, -42.4143)
  arc A272 (-30.7338, -61.4643) -> (-30.2338, -61.9643) centre (-30.2338, -61.4643) ccw
  line L264 (-30.7338, -61.4643) -> (-30.7338, -48.4643)
  arc A273 (-30.2338, -47.9643) -> (-30.7338, -48.4643) centre (-30.2338, -48.4643) ccw
  line L265 (-30.2338, -47.9643) -> (-17.2338, -47.9643)
  arc A274 (-16.7338, -48.4643) -> (-17.2338, -47.9643) centre (-17.2338, -48.4643) ccw
  line L266 (-16.7338, -48.4643) -> (-16.7338, -61.4643)
  arc A275 (-17.2338, -61.9643) -> (-16.7338, -61.4643) centre (-17.2338, -61.4643) ccw
  line L267 (-17.2338, -61.9643) -> (-30.2338, -61.9643)
  arc A276 (-37.4343, -41.9143) -> (-36.9343, -41.4143) centre (-37.4343, -41.4143) ccw
  line L268 (-37.4343, -41.9143) -> (-43.4343, -41.9143)
  arc A277 (-43.9343, -41.4143) -> (-43.4343, -41.9143) centre (-43.4343, -41.4143) ccw
  line L269 (-43.9343, -41.4143) -> (-43.9343, -27.4143)
  arc A278 (-43.4343, -26.9143) -> (-43.9343, -27.4143) centre (-43.4343, -27.4143) ccw
  line L270 (-43.4343, -26.9143) -> (-37.4343, -26.9143)
  arc A279 (-36.9343, -27.4143) -> (-37.4343, -26.9143) centre (-37.4343, -27.4143) ccw
  line L271 (-36.9343, -27.4143) -> (-36.9343, -41.4143)
  arc A280 (-147.4151, -80.5143) -> (-146.9151, -81.0143) centre (-146.9151, -80.5143) ccw
  line L272 (-147.4151, -80.5143) -> (-147.4151, -67.5143)
  arc A281 (-146.9151, -67.0143) -> (-147.4151, -67.5143) centre (-146.9151, -67.5143) ccw
  line L273 (-146.9151, -67.0143) -> (-133.9151, -67.0143)
  arc A282 (-133.4151, -67.5143) -> (-133.9151, -67.0143) centre (-133.9151, -67.5143) ccw
  line L274 (-133.4151, -67.5143) -> (-133.4151, -80.5143)
  arc A283 (-133.9151, -81.0143) -> (-133.4151, -80.5143) centre (-133.9151, -80.5143) ccw
  line L275 (-133.9151, -81.0143) -> (-146.9151, -81.0143)
  arc A284 (-138.6776, -61.9643) -> (-138.1776, -61.4643) centre (-138.6776, -61.4643) ccw
  line L276 (-138.6776, -61.9643) -> (-151.6776, -61.9643)
  arc A285 (-152.1776, -61.4643) -> (-151.6776, -61.9643) centre (-151.6776, -61.4643) ccw
  line L277 (-152.1776, -61.4643) -> (-152.1776, -48.4643)
  arc A286 (-151.6776, -47.9643) -> (-152.1776, -48.4643) centre (-151.6776, -48.4643) ccw
  line L278 (-151.6776, -47.9643) -> (-138.6776, -47.9643)
  arc A287 (-138.1776, -48.4643) -> (-138.6776, -47.9643) centre (-138.6776, -48.4643) ccw
  line L279 (-138.1776, -48.4643) -> (-138.1776, -61.4643)
  arc A288 (-267.2651, -100.0643) -> (-266.7651, -99.5643) centre (-267.2651, -99.5643) ccw
  line L280 (-267.2651, -100.0643) -> (-280.2651, -100.0643)
  arc A289 (-280.7651, -99.5643) -> (-280.2651, -100.0643) centre (-280.2651, -99.5643) ccw
  line L281 (-280.7651, -99.5643) -> (-280.7651, -86.5643)
  arc A290 (-280.2651, -86.0643) -> (-280.7651, -86.5643) centre (-280.2651, -86.5643) ccw
  line L282 (-280.2651, -86.0643) -> (-267.2651, -86.0643)
  arc A291 (-266.7651, -86.5643) -> (-267.2651, -86.0643) centre (-267.2651, -86.5643) ccw
  line L283 (-266.7651, -86.5643) -> (-266.7651, -99.5643)
  arc A292 (-95.8151, -81.0143) -> (-95.3151, -80.5143) centre (-95.8151, -80.5143) ccw
  line L284 (-95.8151, -81.0143) -> (-108.8151, -81.0143)
  arc A293 (-109.3151, -80.5143) -> (-108.8151, -81.0143) centre (-108.8151, -80.5143) ccw
  line L285 (-109.3151, -80.5143) -> (-109.3151, -67.5143)
  arc A294 (-108.8151, -67.0143) -> (-109.3151, -67.5143) centre (-108.8151, -67.5143) ccw
  line L286 (-108.8151, -67.0143) -> (-95.8151, -67.0143)
  arc A295 (-95.3151, -67.5143) -> (-95.8151, -67.0143) centre (-95.8151, -67.5143) ccw
  line L287 (-95.3151, -67.5143) -> (-95.3151, -80.5143)
  arc A296 (-258.8271, -99.0643) -> (-258.3271, -98.5643) centre (-258.8271, -98.5643) ccw
  line L288 (-258.8271, -99.0643) -> (-264.8271, -99.0643)
  arc A297 (-265.3271, -98.5643) -> (-264.8271, -99.0643) centre (-264.8271, -98.5643) ccw
  line L289 (-265.3271, -98.5643) -> (-265.3271, -84.5643)
  arc A298 (-264.8271, -84.0643) -> (-265.3271, -84.5643) centre (-264.8271, -84.5643) ccw
  line L290 (-264.8271, -84.0643) -> (-258.8271, -84.0643)
  arc A299 (-258.3271, -84.5643) -> (-258.8271, -84.0643) centre (-258.8271, -84.5643) ccw
  line L291 (-258.3271, -84.5643) -> (-258.3271, -98.5643)
  arc A300 (-252.1901, -99.5643) -> (-251.6901, -100.0643) centre (-251.6901, -99.5643) ccw
  line L292 (-252.1901, -99.5643) -> (-252.1901, -86.5643)
  arc A301 (-251.6901, -86.0643) -> (-252.1901, -86.5643) centre (-251.6901, -86.5643) ccw
  line L293 (-251.6901, -86.0643) -> (-238.6901, -86.0643)
  arc A302 (-238.1901, -86.5643) -> (-238.6901, -86.0643) centre (-238.6901, -86.5643) ccw
  line L294 (-238.1901, -86.5643) -> (-238.1901, -99.5643)
  arc A303 (-238.6901, -100.0643) -> (-238.1901, -99.5643) centre (-238.6901, -99.5643) ccw
  line L295 (-238.6901, -100.0643) -> (-251.6901, -100.0643)
  arc A304 (-318.8961, -106.6193) -> (-315.8961, -109.6193) centre (-315.8961, -106.6193) ccw
  line L296 (-315.8961, -109.6193) -> (-3.0951, -109.6193)
  arc A305 (-3.0951, -109.6193) -> (-0.0951, -106.6193) centre (-3.0951, -106.6193) ccw
  line L297 (-0.0951, -106.6193) -> (-0.0951, -3.3693)
  arc A306 (-0.0951, -3.3693) -> (-3.0951, -0.3693) centre (-3.0951, -3.3693) ccw
  line L298 (-3.0951, -0.3693) -> (-315.8961, -0.3693)
  arc A307 (-315.8961, -0.3693) -> (-318.8961, -3.3693) centre (-315.8961, -3.3693) ccw
  line L299 (-318.8961, -3.3693) -> (-318.8961, -106.6193)
sketch "草图58" plane through (0, 11, 0) normal (0, 1, 0) x (-1, 0, 0)
  arc A0 (-152.995, -103.62) -> (-153.995, -104.62) centre (-152.995, -104.62) ccw
  line L0 (-153.995, -104.62) -> (-153.995, -109.619)
  line L1 (-153.995, -109.619) -> (-3.0951, -109.619)
  arc A1 (-3.0951, -109.619) -> (-0.0951, -106.619) centre (-3.0951, -106.619) ccw
  line L2 (-0.0951, -106.619) -> (-0.0951, -3.3693)
  arc A2 (-0.0951, -3.3693) -> (-3.0951, -0.3693) centre (-3.0951, -3.3693) ccw
  line L3 (-3.0951, -0.3693) -> (-315.896, -0.3693)
  arc A3 (-315.896, -0.3693) -> (-318.896, -3.3693) centre (-315.896, -3.3693) ccw
  line L4 (-318.896, -3.3693) -> (-318.896, -106.619)
  arc A4 (-318.896, -106.619) -> (-315.896, -109.619) centre (-315.896, -106.619) ccw
  line L5 (-315.896, -109.619) -> (-164.995, -109.619)
  line L6 (-164.995, -109.619) -> (-164.995, -104.62)
  arc A5 (-164.995, -104.62) -> (-165.995, -103.62) centre (-165.995, -104.62) ccw
  line L7 (-165.995, -103.62) -> (-310.395, -103.62)
  arc A6 (-312.895, -101.12) -> (-310.395, -103.62) centre (-310.395, -101.12) ccw
  line L8 (-312.895, -101.12) -> (-312.895, -8.8697)
  arc A7 (-310.395, -6.3697) -> (-312.895, -8.8697) centre (-310.395, -8.8697) ccw
  line L9 (-310.395, -6.3697) -> (-8.5941, -6.3697)
  arc A8 (-6.0942, -8.8697) -> (-8.5941, -6.3697) centre (-8.5942, -8.8697) ccw
  line L10 (-6.0942, -8.8697) -> (-6.0942, -101.12)
  arc A9 (-8.5942, -103.62) -> (-6.0942, -101.12) centre (-8.5942, -101.12) ccw
  line L11 (-8.5942, -103.62) -> (-152.995, -103.62)
  circle A10 centre (-311.895, -3.8697) radius 1.7
  circle A11 centre (-109.895, -3.8697) radius 1.7
  circle A12 centre (-7.0941, -106.12) radius 1.7
  circle A13 centre (-7.0941, -3.8697) radius 1.7
  circle A14 centre (-210.895, -3.8697) radius 1.7
  circle A15 centre (-311.895, -106.12) radius 1.7
  circle A16 centre (-109.895, -106.12) radius 1.7
  circle A17 centre (-210.895, -106.12) radius 1.7
sketch "草图59" plane through (0, 0, 0) normal (0, -1, 0) x (1, 0, 0)
  circle A0 centre (109.895, -106.12) radius 1.7
  circle A1 centre (210.895, -106.12) radius 1.7
  circle A2 centre (311.895, -106.12) radius 1.1
  circle A3 centre (109.895, -3.8697) radius 1.1
  circle A4 centre (7.0941, -106.12) radius 1.1
  circle A5 centre (7.0941, -3.8697) radius 1.1
  circle A6 centre (210.895, -3.8697) radius 1.1
  circle A7 centre (311.895, -3.8697) radius 1.1
  arc A8 (3.0951, -0.3693) -> (0.0951, -3.3693) centre (3.0951, -3.3693) ccw
  line L0 (0.0951, -3.3693) -> (0.0951, -106.619)
  arc A9 (0.0951, -106.619) -> (3.0951, -109.619) centre (3.0951, -106.619) ccw
  line L1 (3.0951, -109.619) -> (315.896, -109.619)
  arc A10 (315.896, -109.619) -> (318.896, -106.619) centre (315.896, -106.619) ccw
  line L2 (318.896, -106.619) -> (318.896, -3.3693)
  arc A11 (318.896, -3.3693) -> (315.896, -0.3693) centre (315.896, -3.3693) ccw
  line L3 (315.896, -0.3693) -> (3.0951, -0.3693)
sketch "草图60" plane through (0, -3, 0) normal (0, -1, 0) x (1, 0, 0)
  arc A0 (23.0951, -84.619) -> (20.0951, -87.619) centre (23.0951, -87.619) ccw
  line L0 (20.0951, -87.619) -> (20.0951, -106.619)
  arc A1 (20.0951, -106.619) -> (23.0951, -109.619) centre (23.0951, -106.619) ccw
  line L1 (23.0951, -109.619) -> (295.896, -109.619)
  arc A2 (295.896, -109.619) -> (298.896, -106.619) centre (295.896, -106.619) ccw
  line L2 (298.896, -106.619) -> (298.896, -87.619)
  arc A3 (298.896, -87.619) -> (295.896, -84.619) centre (295.896, -87.619) ccw
  line L3 (295.896, -84.619) -> (23.0951, -84.619)
  circle A4 centre (109.895, -106.12) radius 1.7
  circle A5 centre (210.895, -106.12) radius 1.7
sketch "草图61" plane through (0, -6, 0) normal (0, -1, 0) x (1, 0, 0)
  arc A0 (23.0951, -89.619) -> (20.0951, -92.619) centre (23.0951, -92.619) ccw
  line L0 (20.0951, -92.619) -> (20.0951, -106.619)
  arc A1 (20.0951, -106.619) -> (23.0951, -109.619) centre (23.0951, -106.619) ccw
  line L1 (23.0951, -109.619) -> (295.896, -109.619)
  arc A2 (295.896, -109.619) -> (298.896, -106.619) centre (295.896, -106.619) ccw
  line L2 (298.896, -106.619) -> (298.896, -92.619)
  arc A3 (298.896, -92.619) -> (295.896, -89.619) centre (295.896, -92.619) ccw
  line L3 (295.896, -89.619) -> (23.0951, -89.619)
  circle A4 centre (109.895, -106.12) radius 1.7
  circle A5 centre (210.895, -106.12) radius 1.7
sketch "草图62" plane through (0, -9, 0) normal (0, -1, 0) x (1, 0, 0)
  arc A0 (23.0951, -94.619) -> (20.0951, -97.619) centre (23.0951, -97.619) ccw
  line L0 (20.0951, -97.619) -> (20.0951, -106.619)
  arc A1 (20.0951, -106.619) -> (23.0951, -109.619) centre (23.0951, -106.619) ccw
  line L1 (23.0951, -109.619) -> (295.896, -109.619)
  arc A2 (295.896, -109.619) -> (298.896, -106.619) centre (295.896, -106.619) ccw
  line L2 (298.896, -106.619) -> (298.896, -97.619)
  arc A3 (298.896, -97.619) -> (295.896, -94.619) centre (295.896, -97.619) ccw
  line L3 (295.896, -94.619) -> (23.0951, -94.619)
  circle A4 centre (109.895, -106.12) radius 1.7
  circle A5 centre (210.895, -106.12) radius 1.7